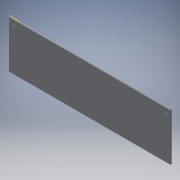
# Autodesk Inventor part: Front.ipt plate
Saved by Autodesk Inventor 2016 (Build 200138000, 138)
## iProperties
Created: 2016-07-16
Part Number: Front.ipt plate
Material: Generic
Document SubType Name: Modeling
Designer: Scott
Density: 1 g/cm^3
Appearance: Default
Author: Scott
Autodesk Inventor part; units mm, degrees
ref_plane "YZ Plane" through (0, 0, 0) normal (1, 0, 0) x (0, 1, 0)
ref_plane "XZ Plane" through (0, 0, 0) normal (0, 1, 0) x (-1, 0, 0)
ref_plane "Work Plane1" through (0, 0, 0) normal (0, 0, 1) x (1, 0, 0)
sketch "Sketch1" plane through (0, 0, 0) normal (0, 0, 1) x (1, 0, 0)
  circle A0 centre (12.7, -12.7) radius 3.175 projected
  line L0 (0, 0) -> (0, -25.4895) projected
  line L1 (25.4, -25.4895) -> (0, -25.4895) projected
  line L2 (25.4, 0) -> (25.4, -25.4895) projected
  line L3 (0, 0) -> (25.4, 0) projected
  line L4 (0, 0) -> (457.2, 0)
  line L5 (457.2, 0) -> (457.2, -133.6856)
  line L6 (457.2, -133.6856) -> (0, -133.6856)
  line L7 (0, -133.6856) -> (0, 0)
  line L8 (457.2, 0) -> (444.5, 0)
  line L9 (444.5, 0) -> (444.5, -12.7)
  circle A1 centre (444.5, -12.7) radius 3.175
  dimension "d0" = 457.2
  dimension "d1" = 12.7
  dimension "d2" = 12.7
  dimension "d3" = 6.35
  constraints: 12 end point, 2 parallel, 1 centre point, 1 coincident, 1 horizontal, 1 perpendicular, 1 point on line, 1 vertical
  measures "d0" distance of L5.end L6.end
  measures "d1" distance of L4.end L8.end
  measures "d2" distance of L8.end L9.end
  measures "d3" diameter of A1
ref_plane "Work Plane2" through (0, -25.4254, 3.81) normal (0, 0, -1) x (0, 1, 0)
extrude "Extrusion1" add sketch "Sketch1" along normal up to surface (3.81 mm away)
body "Solid1"
